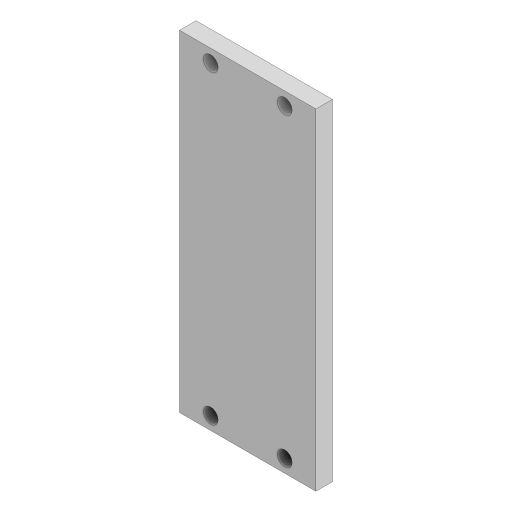
# Autodesk Inventor part: PicoTest
Saved by Autodesk Inventor 2023 (Build 270158000, 158)
## iProperties
Created: 2022-10-31
Part Number: PicoTest
Material: Generic
Document SubType Name: Modeling
Designer: Kyler Martinez
Density: 1 g/cm^3
Appearance: Default
Author: Kyler Martinez
Autodesk Inventor part; units mm, degrees
ref_plane "YZ Plane" through (0, 0, 0) normal (1, 0, 0) x (0, 1, 0)
ref_plane "XZ Plane" through (0, 0, 0) normal (0, 1, 0) x (-1, 0, 0)
ref_plane "XY Plane" through (0, 0, 0) normal (0, 0, 1) x (1, 0, 0)
sketch "Sketch1" plane through (0, 0, 0) normal (0, 0, 1) x (1, 0, 0)
  line L0 (-8.0405, 16.8694) -> (12.9595, 16.8694)
  line L1 (12.9595, 16.8694) -> (12.9595, -34.1306)
  line L2 (12.9595, -34.1306) -> (-8.0405, -34.1306)
  line L3 (-8.0405, -34.1306) -> (-8.0405, 16.8694)
  circle A0 centre (-3.2405, 14.8694) radius 1.05
  circle A1 centre (8.1595, 14.8694) radius 1.05
  circle A2 centre (-3.2405, -32.1306) radius 1.05
  circle A3 centre (8.1595, -32.1306) radius 1.05
  circle A4 centre (-3.2405, 14.8694) radius 1.15
  circle A5 centre (8.1595, 14.8694) radius 1.15
  circle A6 centre (-3.2405, -32.1306) radius 1.15
  circle A7 centre (8.1595, -32.1306) radius 1.15
  point P0 (0, 0)
  dimension "d0" = 21
  dimension "d1" = 51
  dimension "d2" = 2.1
  dimension "d3" = 2.1
  dimension "d4" = 2.1
  dimension "d5" = 2.1
  dimension "d6" = 2
  dimension "d7" = 2
  dimension "d8" = 2
  dimension "d9" = 2
  dimension "d10" = 11.4
  dimension "d11" = 4.8
  dimension "d12" = 11.4
  dimension "d13" = 4.8
  dimension "d14" = 0.1
  dimension "d15" = 0.1
  dimension "d16" = 0.1
  dimension "d17" = 0.1
  constraints: 8 centre point, 8 end point, 2 parallel, 1 horizontal, 1 perpendicular
  measures "d0" distance of L0.start L0.end
  measures "d1" distance of L0.end L1.end
  measures "d2" diameter of A0
  measures "d3" diameter of A1
  measures "d4" diameter of A3
  measures "d5" diameter of A2
  measures "d6" distance from line of A0.centre L0
  measures "d7" distance from line of A1.centre L0
  measures "d8" distance from line of L2 A3.centre
  measures "d9" distance from line of L2 A2.centre
  measures "d10" distance of A1.centre A0.centre
  measures "d11" distance from line of L3 A0.centre
  measures "d12" distance of A3.centre A2.centre
  measures "d13" distance from line of L1 A3.centre
  measures "d14" radial gap between concentric circles of A0 A4
  measures "d15" radial gap between concentric circles of A1 A5
  measures "d16" radial gap between concentric circles of A2 A6
  measures "d17" radial gap between concentric circles of A3 A7
extrude "Extrusion1" add sketch "Sketch1" along normal blind 2.54 contours L0 L1 L2 L3
body "Solid1"
